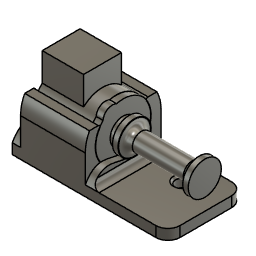
StepperBalls v39 (Autodesk Fusion 360 design; units mm, degrees)
Autodesk Fusion 360 part; units mm, degrees
sketch "Sketch1" plane through (0, 0, 0) normal (1, 0, 0) x (0, 0, -1) in component "motor"
  circle A0 centre (0, 0) radius 4
  dimension "d1" = 8
  constraint coincident A0.centre origin
  measures "d1" diameter of A0
extrude "Extrude1" add sketch "Sketch1" along normal blind 9 makes body 1 in component "motor"
sketch "Sketch2" plane through (9, 0, 0) normal (1, 0, 0) x (0, 0, -1) in component "motor"
  circle A0 centre (0, 0) radius 4
  circle A1 centre (0, 0) radius 1.9
  dimension "d4" = 3.8
  constraint concentric A0 A1
  measures "d4" diameter of A1
extrude "Extrude2" add sketch "Sketch2" along normal blind 0.75 contours A1 bodies 1 in component "motor"
sketch "Sketch3" plane through (9.75, 0, 0) normal (1, 0, 0) x (0, 0, -1) in component "motor"
  circle A0 centre (0, 0) radius 1.9
  circle A1 centre (0, 0) radius 0.4
  dimension "d7" = 0.8
  constraint concentric A0 A1
  measures "d7" diameter of A1
extrude "Extrude3" add sketch "Sketch3" along normal blind 3.5 contours A1 bodies 1 in component "motor"
ref_plane "WorkPlane1" through (0, 0, 0) normal (0, 1, 0) x (0, 0, 1) in component "motor"
sketch "Sketch4" plane through (0, 0, 0) normal (0, 1, 0) x (1, 0, 0) in component "motor"
  line L0 (0, 2.75) -> (6, 2.75)
  line L1 (6, 2.75) -> (6, -2.75)
  line L2 (6, -2.75) -> (0, -2.75)
  line L3 (0, -2.75) -> (0, 2.75)
  line L4 (1.75, 0) -> (22.5, 0)
  dimension "d11" = 6
  dimension "d12" = 5.5
  constraint horizontal L0
  constraint vertical L1
  constraint horizontal L2
  constraint vertical L3
  constraint symmetric L0 L2 L4
  measures "d11" distance of L0.start L0.end
  measures "d12" distance of L0.start L2.end
extrude "Extrude4" add sketch "Sketch4" along normal blind 7 bodies 1 in component "motor"
sketch "Sketch5" plane through (9, 0, 0) normal (1, 0, 0) x (0, 0, -1) in component "motor"
  circle A0 centre (0, 0) radius 1.9
  circle A1 centre (0, 0) radius 4
  circle A2 centre (0, 0) radius 4.5
  dimension "d23" = 9
  constraint coincident A0.centre A1.centre
  measures "d23" diameter of A2
extrude "Extrude5" add sketch "Sketch5" against normal blind 1 contours A2 bodies 1 in component "motor"
sketch "Sketch7" plane through (9, 0, 0) normal (1, 0, 0) x (0, 0, -1) in component "motor"
  circle A0 centre (0, 0) radius 4.5
  circle A1 centre (0, 0) radius 1.9
  circle A2 centre (0, 0) radius 4
  line L0 (-2.7743, 4.8052) -> (2.547, -4.4116) construction
  circle A3 centre (-1.575, 2.728) radius 1.35
  circle A4 centre (1.575, -2.728) radius 1.35
  circle A5 centre (0, 0) radius 4.05
  line L1 (0, 0) -> (-5.4331, 0) construction
  dimension "d84" = 2.7
  dimension "d87" = 0.05
  dimension "d133" = 60
  constraint coincident A0.centre L0
  constraint coincident L0 A3.centre
  constraint tangent A0 A3
  constraint coincident L0 A4.centre
  constraint tangent A0 A4
  constraint equal A3 A4
  constraint coincident A0.centre A1.centre
  constraint horizontal L1
  measures "d84" diameter of A3
  measures "d133" angle of L0 L1
extrude "Extrude8" cut sketch "Sketch7" against normal up to surface (1 mm away) contours A0 A3 A4 A5 | A0 A3 A4 A5 bodies 1 in component "motor"
sketch "Sketch2 (2)" plane through (9, 0, 0) normal (1, 0, 0) x (0, 0, -1) in component "mount"
  circle A0 centre (0, 0) radius 4
  circle A1 centre (0, 0) radius 5.5
  line L0 (-5.5, 2.5) -> (5.5, 2.5)
  line L1 (5.5, 2.5) -> (5.5, -5.5)
  line L2 (5.5, -5.5) -> (-5.5, -5.5)
  line L3 (-5.5, -5.5) -> (-5.5, 2.5)
  circle A2 centre (0, 0) radius 4
  circle A3 centre (0, 0) radius 4.5
  circle A4 centre (0, 0) radius 1.9
  arc A5 (0.9664, -3.933) -> (2.9229, -2.8034) centre (1.575, -2.728) ccw
  arc A6 (2.9229, -2.8034) -> (-0.9664, 3.933) centre (0, 0) ccw
  arc A7 (-0.9664, 3.933) -> (-2.9229, 2.8034) centre (-1.575, 2.728) ccw
  arc A8 (-2.9229, 2.8034) -> (0.9664, -3.933) centre (0, 0) ccw
  dimension "d18" = 1.5
  dimension "d20" = 2.5
  constraint horizontal L0
  constraint vertical L1
  constraint horizontal L2
  constraint vertical L3
  constraint tangent A1 L2
  constraint tangent A1 L1
  constraint tangent A1 L3
  measures "d20" distance of A0.centre L0
extrude "Extrude1'" add sketch "Sketch2 (2)" against normal blind 9.4 separate body contours A0 L0 A2 A5 A6 A8 | L0 A3 A5 A6 | L0 A3 A5 A8 | A1 L0 A3 | A1 L1 L2 | A1 L2 L3 picked at (-0.3699, -5.144) makes body 2 in component "mount"
sketch "Sketch4 (2)" plane through (9, 0, 0) normal (1, 0, 0) x (0, 0, -1) in component "mount"
  line L0 (-2.4678, -4) -> (-5.5, -4)
  line L1 (-5.5, -4) -> (-5.5, -5.5)
  line L2 (-5.5, -5.5) -> (5.5, -5.5)
  line L3 (5.5, -5.5) -> (5.5, -4)
  line L4 (5.5, -4) -> (2.4678, -4)
  line L5 (-5.5, -5.5) -> (5.5, -5.5)
  line L6 (5.5, -5.5) -> (5.5, -4)
  line L7 (5.5, -4) -> (-5.5, -4)
  line L8 (-5.5, -4) -> (-5.5, -5.5)
  line L9 (-5.5, 0) -> (-5.5, -5.5)
  line L10 (-5.5, -5.5) -> (5.5, -5.5)
  line L11 (5.5, -5.5) -> (5.5, 0)
  line L12 (4.899, 2.5) -> (3.1225, 2.5)
  arc A0 (-3.1225, 2.5) -> (3.1225, 2.5) centre (0, 0) ccw
  arc A1 (-4.899, 2.5) -> (-5.5, 0) centre (0, 0) ccw
  arc A2 (5.5, 0) -> (4.899, 2.5) centre (0, 0) ccw
  line L13 (-3.1225, 2.5) -> (-4.899, 2.5)
  constraint horizontal L5
  constraint vertical L6
  constraint horizontal L7
  constraint vertical L8
  constraint coincident L3.end L4.start
  constraint coincident L1.end L2.start
extrude "Extrude3'" add sketch "Sketch4 (2)" along normal blind 10 contours L0 L1 L2 L3 L4 L5 L6 L7 L8 L9 L10 L11 bodies 2 in component "mount"
sketch "Sketch5 (2)" plane through (19, 0, 0) normal (1, 0, 0) x (0, 0, -1) in component "mount"
  line L0 (-5.5, -5.5) -> (5.5, -5.5)
  line L1 (-5.5, -5.5) -> (-5.5, 0)
  line L2 (5.5, 0) -> (5.5, -5.5)
  circle A0 centre (0, -1.6771) radius 5.75
  ellipse E0 centre (0, 0.2) end of major axis (2.05, 0.2) minor radius 2.15
  line L3 (-2.05, 0.2) -> (2.05, 0.2) construction
  line L4 (0, -1.95) -> (0, 2.35) construction
  dimension "d110" = 4.1
  dimension "d111" = 4.3
  dimension "d122" = 11.5
  dimension "d123" = 0.2
  constraint coincident L1.end A0
  constraint coincident L2.start A0
  constraint coincident E0 L3.start
  constraint coincident E0 L3.end
  constraint coincident E0 L4.start
  constraint coincident E0 L4.end
  constraint horizontal L3
  constraint vertical origin E0.centre
  measures "d110" distance of E0
  measures "d122" diameter of A0
  measures "d123" distance of origin E0.centre
extrude "Extrude4'" add sketch "Sketch5 (2)" along normal blind 2 contours L0 L1 A0 | L0 L1 L2 A0 | L0 L2 A0 bodies 2 in component "mount"
sketch "Sketch6" plane through (0, -4, 0) normal (0, 1, 0) x (-1, 0, 0) in component "mount"
  line L0 (-9, 5.5) -> (-19, 5.5)
  line L1 (-19, 5.5) -> (-19, -5.5)
  line L2 (-19, -5.5) -> (-9, -5.5)
  line L3 (-1.75, 0) -> (-22.5, 0)
  circle A0 centre (-15.6174, -1.9924) radius 1
  line L4 (-9, -5.5) -> (-9, 0)
  line L5 (-9, 0) -> (-9, 5.5)
  dimension "d47" = 2
  measures "d47" diameter of A0
extrude "Extrude5'" cut sketch "Sketch6" against normal through all contours A0 bodies 2 in component "mount"
sketch "Sketch6 (2)" plane through (13.25, 0, 0) normal (1, 0, 0) x (0, 0, -1) in component "motor"
  circle A0 centre (0, 0) radius 0.4
  circle A1 centre (0, 0) radius 1.14
  dimension "d38" = 2.28
  constraint coincident A0.centre A1.centre
  measures "d38" diameter of A1
extrude "Extrude6" add sketch "Sketch6 (2)" against normal blind 1.3 bodies 1 in component "motor"
sketch "Sketch11" plane through (9, 0, 0) normal (1, 0, 0) x (0, 0, -1) in component "mount"
  line L0 (-5.5, -4) -> (5.5, -4)
  spline S0 degree 5 poles (-5.5, -4) (-5.4153, -3.8522) (-5.243, -3.5725) (-4.9763, -3.2006) (-4.6039, -2.8004) (-4.1104, -2.459) (-3.5888, -2.2709) (-3.0401, -2.2217) (-2.4661, -2.2841) (-1.8702, -2.4139) (-1.2569, -2.5598) (-0.6315, -2.6728) (0, -2.7157) (0.6315, -2.6728) (1.2569, -2.5598) (1.8702, -2.4139) (2.4661, -2.2841) (3.0401, -2.2217) (3.5888, -2.2709) (4.1104, -2.459) (4.6039, -2.8004) (4.9763, -3.2006) (5.243, -3.5725) (5.4153, -3.8522) (5.5, -4) knots 0 0 0 0 0 0 0.05 0.1 0.15 0.2 0.25 0.3 0.35 0.4 0.45 0.5 0.55 0.6 0.65 0.7 0.75 0.8 0.85 0.9 0.95 1 1 1 1 1 1
  line L1 (0, 0) -> (0, -4.65) construction
  point P0 (-5.5, -4)
  point P1 (5.5, -4)
  point P2 (-3.0464, -2.2494)
  point P3 (0, -2.6945)
  point P4 (3.0464, -2.2494)
  constraint coincident P0 L0.start
  constraint coincident P1 L0.end
  constraint coincident L1.start origin
  constraint perpendicular L0 L1
  constraint horizontal P2 P4
  constraint symmetric P2 P4 L1
  constraint coincident P3 L1
extrude "Extrude12" add sketch "Sketch11" along normal blind 1 bodies 2 in component "mount"
sketch "Sketch1 (2)" plane through (9, 0, 0) normal (-1, 0, 0) x (0, 0, 1)
  arc A0 (-3.1225, 2.5) -> (3.1225, 2.5) centre (0, 0) ccw
  arc A1 (-2.9229, -2.8034) -> (-0.9664, -3.933) centre (-1.575, -2.728) ccw
  line L0 (-2.9229, -2.8034) -> (-0.9664, -3.933)
  line L1 (-0.9664, -3.933) -> (0.9416, -0.6283)
  line L2 (0.9416, -0.6283) -> (-1.0149, 0.5013)
  line L3 (-1.0149, 0.5013) -> (-2.9229, -2.8034)
  line L4 (0, 0) -> (0, -5.7471) construction
  arc A2 (0.9664, -3.933) -> (2.9229, -2.8034) centre (1.575, -2.728) ccw
  line L5 (1.0149, 0.5013) -> (2.9229, -2.8034)
  line L6 (0.9664, -3.933) -> (-0.9416, -0.6283)
  constraint perpendicular L0 L1
  constraint parallel L0 L2
  constraint parallel L1 L3
  constraint coincident A1.end L0.end
  constraint coincident A1.start L0.start
  constraint coincident A0.centre L4.start
  constraint vertical L4
  constraint symmetric A1.start L4 A2.end
  constraint symmetric A1.end L4 A2.start
  constraint symmetric A1 L4 A2
  constraint symmetric L1.end L4 L6.end
  constraint symmetric L2.end L4 L5.start
sketch "Sketch13" plane through (-0.4, 0, 0) normal (-1, 0, 0) x (0, 0, 1) in component "mount"
  line L0 (-5.5, -5.5) -> (5.5, -5.5)
  line L1 (5.5, -5.5) -> (5.5, 0)
  line L2 (-5.5, 0) -> (-5.5, -5.5)
  line L3 (-5.5, -4) -> (5.5, -4)
  spline S0 degree 5 poles (-5.5, -4) (-5.4153, -3.8522) (-5.243, -3.5725) (-4.9763, -3.2006) (-4.6039, -2.8004) (-4.1104, -2.459) (-3.5888, -2.2709) (-3.0401, -2.2217) (-2.4661, -2.2841) (-1.8702, -2.4139) (-1.2569, -2.5598) (-0.6315, -2.6728) (0, -2.7157) (0.6315, -2.6728) (1.2569, -2.5598) (1.8702, -2.4139) (2.4661, -2.2841) (3.0401, -2.2217) (3.5888, -2.2709) (4.1104, -2.459) (4.6039, -2.8004) (4.9763, -3.2006) (5.243, -3.5725) (5.4153, -3.8522) (5.5, -4) knots -1 -1 -1 -1 -1 -1 -0.95 -0.9 -0.85 -0.8 -0.75 -0.7 -0.65 -0.6 -0.55 -0.5 -0.45 -0.4 -0.35 -0.3 -0.25 -0.2 -0.15 -0.1 -0.05 0 0 0 0 0 0
extrude "Extrude16" add sketch "Sketch13" along normal blind 1.2 bodies 2 in component "mount"
sketch "Sketch17" plane through (9, 0, 0) normal (-1, 0, 0) x (0, 0, 1) in component "mount"
  arc A0 (-2.9229, -2.8034) -> (-0.9664, -3.933) centre (-1.575, -2.728) ccw
  arc A1 (-2.9229, -2.8034) -> (-0.9664, -3.933) centre (-1.575, -2.728) ccw
  line L0 (0, 0) -> (0, 1.9136) construction
  circle A2 centre (-1.575, -2.728) radius 1.4
  circle A3 centre (1.575, -2.728) radius 1.4
  point P0 (-2.9229, -2.8034)
  point P1 (-0.9664, -3.933)
  dimension "d128" = 2.8
  constraint coincident L0.start origin
  constraint vertical L0
  constraint concentric A0 A2
  constraint symmetric L0 A2 A3
  measures "d128" diameter of A2
extrude "Extrude22" cut sketch "Sketch17" along normal blind 1.1 bodies 2 in component "mount"
fillet "Fillet10" radius 2.1 5 edges at (8.45, -3.913, 0.8296) (8.45, -2.6749, 2.974) (8.45, -3.913, 0.8296) (8.45, -2.6749, -2.974) (8.45, -2.6749, -2.974) on bodies 2 in component "mount"
fillet "Fillet11" radius 1 2 edges at (19, -4, 0) (10, -4, 0) on bodies 2 in component "mount"
fillet "Fillet12" radius 0.25 3 edges at (4.3, 2.5, 3.1225) (4.3, 2.5, -3.1225) (4.3, 2.5, -3.1225) on bodies 2 in component "mount"
sketch "Sketch1 (3)" plane through (0, 0, 0) normal (1, 0, 0) x (0, 0, -1) in component "shaft (1)"
  circle A0 centre (0, 1.4801) radius 0.315
  line L0 (0.515, 11) -> (2.4, 11)
  line L1 (0, 11) -> (0, 0)
  line L2 (0.515, 0) -> (2.4, 0)
  line L3 (0, 0) -> (0.515, 0)
  line L4 (0.515, 11) -> (0, 11)
  line L5 (0.515, 0) -> (0.515, 11)
  line L6 (0.515, 6.5) -> (0, 6.5)
  line L7 (2.4, 11) -> (2.4, 10.2)
  line L8 (2.4, 0) -> (2.4, 0.8)
  line L9 (2.4, 10.2) -> (1.315, 10.2)
  line L10 (1.315, 10.2) -> (1.315, 0.8)
  line L11 (1.315, 0.8) -> (2.4, 0.8)
  dimension "d138" = 0.515
  dimension "d139" = 11
  dimension "d142" = 2.4
  dimension "d143" = 0.63
  dimension "d158" = 4.5
  dimension "d160" = 0.8
  dimension "d161" = 0.8
  dimension "d162" = 0.8
  constraint horizontal L3
  constraint vertical L5
  constraint horizontal L4
  constraint vertical L1
  constraint coincident L1.end L3.start
  constraint perpendicular L2 L5
  constraint perpendicular L0 L5
  constraint equal L0 L2
  constraint coincident L5 L6.start
  constraint coincident L1 L6.end
  constraint perpendicular L1 L6
  constraint perpendicular L0 L7
  constraint perpendicular L2 L8
  constraint perpendicular L7 L9
  constraint perpendicular L9 L10
  constraint perpendicular L8 L11
  constraint coincident A0.centre L1
  measures "d138" distance of L2.start L1.end
  measures "d139" distance of L1.start L1.end
  measures "d142" distance of L2.end L1.end
  measures "d143" diameter of A0
  measures "d158" distance of L4 L6
  measures "d160" distance of L0.end L7.end
  measures "d161" distance of L2.end L8.end
  measures "d162" distance of L5 L10
revolve "Revolve1" add sketch "Sketch1 (3)" angle 360 about axis through (0, 11, 0) along (0, -1, 0) separate body contours A0 L1 | A0 L1 L3 L5 L6 | L0 L2 L5 L7 L8 L9 L10 L11 picked at (0.0794, 1.5488) makes body 3 in component "shaft (1)"
chamfer "Chamfer1" distance 0.1 distance2 0.3 1 edges at (-0.4801, 11, -0.1862) measured on face at (-0.1192, 11, -1.7627) on bodies 3 in component "shaft (1)"
sketch "Sketch18" plane through (0, -4, 0) normal (0, 1, 0) x (-1, 0, 0) in component "mount"
  line L0 (-11, -5.5) -> (-11, 5.5)
  line L1 (-11, 5.5) -> (-18, 5.5)
  line L2 (-18, 5.5) -> (-18, -5.5)
  line L3 (-18, -5.5) -> (-11, -5.5)
  circle A0 centre (-15.6174, -1.9924) radius 1
  line L4 (-17.3183, -5.5) -> (-22.1168, -5.5)
  line L5 (-22.1168, -5.5) -> (-22.1168, 5.5)
  line L6 (-22.1168, 5.5) -> (-17.3183, 5.5)
  line L7 (-17.3183, 5.5) -> (-17.3183, -5.5)
  constraint horizontal L4
  constraint vertical L5
  constraint horizontal L6
  constraint vertical L7
  constraint coincident L3 L4.start
extrude "Extrude23" cut sketch "Sketch18" along normal through all contours L1 L2 L3 L4 L6 L7 | L2 L4 L5 L6 bodies 2 in component "mount"
fillet "Fillet13" radius 1.75 2 edges at (21, -4.75, 5.5) (21, -4.75, -5.5) on bodies 2 in component "mount"
fillet "Fillet2" radius 1 2 edges at (-1.226, 10.2, -0.4755) (-1.226, 0.8, -0.4755) on bodies 3 in component "shaft (1)"
extrude "Extrude1''" cut sketch "Sketch1 (3)" along normal through all and the other way through all contours A0 L1 | A0 L1 bodies 3 in component "shaft (1)"
chamfer "Chamfer5" distance 0.3 angle 45 1 edges at (16.5497, -4, -1.6308) on bodies 2 in component "mount"
component "motor" placed x (1, 0, 0) y (0, 1, 0) z (0, 0, 1) at (0, 0, 0)
component "mount" placed x (1, 0, 0) y (0, 1, 0) z (0, 0, 1) at (0, 0, 0)
component "shaft (1)" placed x (0, -1, 0) y (-1, 0, 0) z (0, 0, -1) at (20.85, 0, 0)
equation "d138 = ( 1.03 / 2 ) * 1 mm"
equation "d142 = ( 4.8 / 2 ) * 1 mm"
